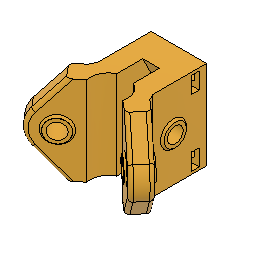
X-Roller v7(1) (Autodesk Fusion 360 design; units mm, degrees)
Autodesk Fusion 360 part; units mm, degrees
note: some values were not read from the file. Chosen so that the rebuilt part matches the saved one: a direction.
sketch "Sketch2" plane through (0, 0, 0) normal (0, 1, 0) x (1, 0, 0) in component "rollers sketches 18mm v10"
  circle A0 centre (0, 0) radius 13.55
  circle A1 centre (0, 0) radius 9.1
  line L0 (0, 0) -> (0, 50) construction
  line L1 (0, 0) -> (38.3022, -32.1394) construction
  line L2 (0, 0) -> (50, 0) construction
  line L3 (0, 0) -> (-38.3022, -32.1394) construction
  line L4 (0, 0) -> (50, 0) construction
  dimension "d20" = 27.1
  dimension "d21" = 18.2
  dimension "d22" = 40
  dimension "d23_1" = 50
  dimension "d24_1" = 140
  dimension "d25_1" = 50
  dimension "d26_1" = 11
  dimension "d27_1" = 11
  dimension "d28_1" = 11
  dimension "d132" = 50
  measures "d20" diameter of A0
  measures "d21" diameter of A1
  measures "d22" angle of L1 L2
  measures "d24_1" angle of L3 L4
  measures "d28_1" distance of A0.centre
sketch "Sketch3" plane through (0, 0, 0) normal (1, 0, 0) x (0, 0, -1) in component "rollers sketches 18mm v10"
  circle A0 centre (20.1, 0) radius 4.2
  circle A1 centre (20.1, 0) radius 11
  circle A2 centre (20.1, 0) radius 6
  circle A3 centre (20.1, 0) radius 13.25
  line L0 (20.1, -13.25) -> (0.1513, -13.25)
  line L1 (20.1, 13.25) -> (0.1513, 13.25)
  line L2 (0.1513, 13.25) -> (0.1513, -13.25)
  line L3 (0.1514, -70) -> (0.1513, 70)
  line L4 (0.1513, 70) -> (31.9687, 5.8904)
  line L5 (0.1514, -70) -> (31.9687, -5.8904)
  dimension "d29_1" = 8.4
  dimension "d30_1" = 22
  dimension "d31_1" = 12
  dimension "d62_1" = 26.5
  dimension "d144" = 70
  dimension "d145" = 70
  measures "d29_1" diameter of A0
  measures "d30_1" diameter of A1
  measures "d31_1" diameter of A2
  measures "d62_1" diameter of A3
ref_plane "WorkPlane1" through (-19.1511, 0, 16.0697) normal (0.642788, 0, 0.766044) x (-0.766044, 0, 0.642788) in component "rollers sketches 18mm v10"
ref_plane "WorkPlane2" through (19.1511, 0, 16.0697) normal (-0.642788, 0, 0.766044) x (0.766044, 0, 0.642788) in component "rollers sketches 18mm v10"
sketch "Sketch4" plane through (-19.1511, 0, 16.0697) normal (0.642788, 0, 0.766044) x (-0.766044, 0, 0.642788) in component "rollers sketches 18mm v10"
  line L0 (23.05, 0) -> (50, 0)
  circle A0 centre (-4.9, 0) radius 4.25
  circle A1 centre (-4.9, 0) radius 6
  circle A2 centre (-4.9, 0) radius 11
  circle A3 centre (-4.9, 0) radius 13.25
  line L1 (-25, 0) -> (-25, 13.25)
  line L2 (-25, 13.25) -> (-4.9, 13.25)
  line L3 (-25, 0) -> (-24.9683, -13.25)
  line L4 (-24.9683, -13.25) -> (-4.9, -13.25)
  line L5 (11.7612, -31.776) -> (-18.2997, -31.776)
  line L6 (-18.2997, -31.776) -> (-18.2997, 33.967)
  line L7 (-18.2997, 33.967) -> (11.7612, 33.967)
  line L8 (11.7612, 33.967) -> (11.7612, -31.776)
  line L9 (-18, 35) -> (-18, -35)
  line L10 (-18, -35) -> (5.0564, -8.7426)
  line L11 (-18, 35) -> (5.0564, 8.7426)
  dimension "d40_1" = 8.5
  dimension "d42_1" = 12
  dimension "d43" = 22
  dimension "d96" = 26.5
  dimension "d139" = 13.25
  dimension "d140" = 13.25
  dimension "d148" = 35
  dimension "d154" = 35
  dimension "d155" = 7
  measures "d40_1" diameter of A0
  measures "d42_1" diameter of A1
  measures "d43" diameter of A2
  measures "d96" diameter of A3
  measures "d139" distance of origin
  measures "d140" distance of origin
  measures "d148" distance of origin
  measures "d154" distance of origin
  measures "d155" distance of L9 origin
sketch "Sketch5" plane through (19.1511, 0, 16.0697) normal (-0.642788, 0, 0.766044) x (0.766044, 0, 0.642788) in component "rollers sketches 18mm v10"
  line L0 (-44.9577, 0) -> (-39.8242, 0)
  circle A0 centre (-4.9, 0) radius 4.25
  circle A1 centre (-4.9, 0) radius 6
  circle A2 centre (-4.9, 0) radius 11
  circle A3 centre (-4.9, 0) radius 13.25
  dimension "d41_1" = 8.5
  dimension "d44" = 12
  dimension "d45" = 22
  dimension "d97" = 26.5
  measures "d41_1" diameter of A0
  measures "d44" diameter of A1
  measures "d45" diameter of A2
  measures "d97" diameter of A3
sketch "Sketch7" plane through (0, 0, 0) normal (0, 1, 0) x (1, 0, 0) in component "rollers sketches 18mm v10"
  circle A0 centre (0, 0) radius 10
  circle A1 centre (0, 0) radius 13.55
  line L0 (0, 9.1) -> (0, 31.1)
  line L1 (-15, 9.0139) -> (-15, 38)
  line L2 (-15, 38) -> (15, 38)
  line L3 (15, 38) -> (15, 9.0139)
  line L4 (-5.1, 9.0139) -> (-15, 9.0139)
  line L5 (5.1, 9.0139) -> (15, 9.0139)
  line L6 (-15, 9.0139) -> (15, 9.0139)
  line L7 (0, 0) -> (0, 50)
  line L8 (-15, 0) -> (-15, 54) construction
  line L9 (0, 0) -> (50, 0)
  line L10 (0, 0) -> (38.3022, -32.1394)
  line L11 (6.7412, -5.6565) -> (16.383, 5.8341)
  line L12 (16.383, 5.8341) -> (35.1894, -9.9463)
  line L13 (35.1894, -9.9463) -> (25.5476, -21.437)
  circle A2 centre (0, 0) radius 17.5
  line L14 (-23.824, -19.9907) -> (-6.971, -5.8494)
  line L15 (-6.0078, -5.0411) -> (-15.6496, 6.4495)
  line L16 (-15.6496, 6.4495) -> (-35.1894, -9.9463)
  line L17 (-36.8084, -30.8859) -> (-57.4533, -48.2091)
  line L18 (0, 0) -> (-38.3022, -32.1394)
  line L19 (-35.1894, -9.9463) -> (-25.5476, -21.437)
  line L20 (-28.5687, -17.8366) -> (-9.7827, -2.0733)
  line L21 (-25.5476, -21.437) -> (-5.2474, -4.4031)
  line L22 (28.5687, -17.8366) -> (9.7827, -2.0733)
  line L23 (5.2474, -4.4031) -> (25.5476, -21.437)
  dimension "d85_1" = 30
  dimension "d86_1" = 15
  dimension "d89_1" = 8.8
  dimension "d91_1" = 15
  dimension "d95" = 15
  dimension "d98" = 4.7
  dimension "d99_1" = 4.7
  dimension "d120" = 35
  dimension "d149" = 20
  dimension "d134" = 38
  measures "d86_1" distance of L1 L7
  measures "d89_1" distance of A0.centre
  measures "d91_1" distance of A0.centre
  measures "d95" distance of A0.centre
  measures "d98" distance of L20 L21
  measures "d99_1" distance of L22 L23
  measures "d120" diameter of A2
  measures "d149" diameter of A0
  measures "d134" distance of L2 A0.centre
ref_plane "WorkPlane5" through (0, 0, -38) normal (0, 0, 1) x (1, 0, 0) in component "rollers sketches 18mm v10"
sketch "Sketch9" plane through (0, 0, -38) normal (0, 0, 1) x (1, 0, 0) in component "rollers sketches 18mm v10"
  circle A0 centre (-10.5, 36) radius 2.25
  circle A1 centre (10.5, 36) radius 2.25
  circle A2 centre (-10.5, -18) radius 2.25
  circle A3 centre (-10.5, -36) radius 2.25
  circle A4 centre (10.5, 18) radius 2.25
  circle A5 centre (10.5, -36) radius 2.25
  circle A6 centre (10.5, -18) radius 2.25
  circle A7 centre (-10.5, 18) radius 2.25
  line L0 (-15, -24) -> (-15, 24)
  line L1 (-10.5, -54) -> (-10.5, -6.4658) construction
  line L2 (-10.5, -16) -> (-10.5, 31.5342) construction
  line L3 (0, 24) -> (15, 24)
  line L4 (10.5, -36) -> (10.5, 11.5342) construction
  line L5 (-10.5, -36) -> (-10.5, 11.5342) construction
  line L6 (10.5, -18) -> (10.5, 29.5342) construction
  line L7 (-10.5, -18) -> (-10.5, 29.5342) construction
  line L8 (15, -24) -> (0, -24)
  line L9 (15, 24) -> (15, -24)
  line L10 (0, 24) -> (0, -24)
  line L11 (-15, 24) -> (0, 24)
  line L12 (-15, -24) -> (0, -24)
  line L13 (10.5, 0) -> (10.5, 47.5342) construction
  line L14 (10.5, -54) -> (10.5, -6.4658) construction
  line L15 (-15, 0) -> (15, 0)
  dimension "d146" = 4.5
  dimension "d147" = 4.5
  dimension "d172" = 24
  dimension "d173" = 18
  dimension "d174" = 18
  dimension "d175" = 18
  dimension "d176" = 18
  dimension "d177" = 48
  dimension "d178" = 18
  dimension "d179" = 18
  dimension "d180" = 18
  dimension "d181" = 18
  measures "d146" diameter of A0
  measures "d147" distance of L0 L2
  measures "d172" distance of L3 L15
  measures "d173" distance of origin
  measures "d175" distance of origin
  measures "d178" distance of origin
  measures "d179" distance of origin
extrude "Extrude16" add sketch "Sketch7" along normal mid plane 48 contours A0 A1 L0 L4 L6 L7 | A0 A1 L4 L6 L15 | A1 L0 L4 L6 L7 A2 | A0 A1 L15 L20 | A1 L4 L6 A2 L15 L16 | L0 L1 L2 L7 A2 | A1 A2 L15 L16 L20 | A2 L16 L19 L20 makes body 1 in component "rollers sketches 18mm v10"
extrude "Extrude17" cut sketch "Sketch4" against normal blind 31 contours A0 bodies 1 in component "rollers sketches 18mm v10"
extrude "Extrude21" add sketch "Sketch4" against normal blind 16 contours A1 bodies 1 in component "rollers sketches 18mm v10"
extrude "Extrude22" cut sketch "Sketch4" against normal blind 3.5 contours A1 bodies 1 in component "rollers sketches 18mm v10"
extrude "Extrude23" cut sketch "Sketch3" along normal mid plane 58 contours A0 bodies 1 in component "rollers sketches 18mm v10"
extrude "Extrude24" cut sketch "Sketch3" along normal mid plane 9 contours A1 | A3 | A3 L1 L3 L4 | A3 L0 L3 L5 | A3 L0 L1 L2 L3 bodies 1 in component "rollers sketches 18mm v10"
extrude "Extrude25" add sketch "Sketch3" against normal blind 16 contours A2 bodies 1 in component "rollers sketches 18mm v10"
extrude "Extrude26" cut sketch "Sketch3" along normal mid plane 7 contours A2 bodies 1 in component "rollers sketches 18mm v10"
extrude "Extrude27" cut sketch "Sketch4" against normal blind 31 contours A3 L5 L7 L8 L10 L11 bodies 1 in component "rollers sketches 18mm v10"
sketch "Sketch9 (2)" plane through (-15, 0, 0) normal (-1, 0, 0) x (0, 0, 1)
  circle A0 centre (-20.1, 0) radius 6
  line L0 (-9.0139, -24) -> (-9.0139, 24)
  line L1 (-9.0139, 24) -> (-38, 24)
  line L2 (-38, 24) -> (-38, -24)
  line L3 (-38, -24) -> (-9.0139, -24)
  line L4 (-47.8567, 18) -> (-16.3238, 18) construction
  line L5 (-52.0724, -18) -> (-19.1904, -18) construction
  line L6 (-30, 13.5) -> (-34, 13.5)
  line L7 (-34, 13.5) -> (-34, 22.5)
  line L8 (-34, 22.5) -> (-30, 22.5)
  line L9 (-30, 22.5) -> (-30, 13.5)
  line L10 (-30, 13.5) -> (-34, 22.5) construction
  line L11 (-34, 13.5) -> (-30, 22.5) construction
  line L12 (-38, -24) -> (-38, 24)
  line L13 (-34, -13.5) -> (-30, -13.5)
  line L14 (-30, -13.5) -> (-30, -22.5)
  line L15 (-30, -22.5) -> (-34, -22.5)
  line L16 (-34, -22.5) -> (-34, -13.5)
  line L17 (-34, -13.5) -> (-30, -22.5) construction
  line L18 (-30, -13.5) -> (-34, -22.5) construction
  dimension "d156" = 4
  dimension "d157" = 4
  dimension "d158" = 9
  dimension "d159" = 4
  dimension "d182" = 4
  dimension "d183" = 9
  measures "d156" distance of L7 L12
  measures "d158" distance of origin
  measures "d159" distance of L12 L16
  measures "d183" distance of origin
extrude "Extrude28" cut sketch "Sketch9 (2)" against normal blind 10 contours L6 L7 L8 L9 | L13 L14 L15 L16 bodies 1 in component "rollers sketches 18mm v10"
extrude "Extrude29" cut sketch "Sketch9" along normal blind 12 contours A2 | A7 bodies 1 in component "rollers sketches 18mm v10"
fillet "Fillet6" radius 2 6 edges at (-27.5348, -16.3713, 3.5234) (-35.1894, 0, 9.9463) (-27.5348, 16.3713, 3.5234) (-20.9141, 16.3713, 11.4136) (-28.5687, 0, 17.8366) (-20.9141, -16.3713, 11.4136) on bodies 1 in component "rollers sketches 18mm v10"
chamfer "Chamfer3" distance 1 angle 45 4 edges at (-20.7541, 2.1697, -2.1664) (-15, -2.1697, -14.506) (-14.1334, -2.1697, 5.7239) (-4.5, -2.1697, -14.506) on bodies 1 in component "rollers sketches 18mm v10"
copy_body "Body->Comp1" bodies 1 removing the originals makes body 2 in component "XRoller alternative US"
mirror "Mirror1" about plane through (0, 0, -10) normal (1, 0, 0) of bodies 2 makes body 3 in component "XRoller alternative US"
combine "Combine1" operation add target body 2 tool bodies 3 in component "XRoller alternative US"
component "rollers sketches 18mm v10" placed x (1, 0, 0) y (0, 1, 0) z (0, 0, 1) at (0, 0, 0)
component "XRoller alternative US" placed x (1, 0, 0) y (0, 1, 0) z (0, 0, 1) at (0, 0, 0) in component "rollers sketches 18mm v10"
equation "d20 = PipeDiameter + 9.3 mm"
equation "d21 = PipeDiameter + 0.4 mm"
equation "d26_1 = BallBearingRadius"
equation "d27_1 = BallBearingRadius"
equation "d28_1 = BallBearingRadius"
equation "d29_1 = BallBInternalR * 2 + 0.4 mm"
equation "d30_1 = BallBearingRadius * 2"
equation "d31_1 = BallBInternalR * 2 + 4 mm"
equation "d40_1 = BallBInternalR * 2 + 0.5 mm"
equation "d42_1 = BallBInternalR * 2 + 4 mm"
equation "d43 = BallBearingRadius * 2"
equation "d62_1 = BallBearingRadius * 2 + 4.5 mm"
equation "d96 = BallBearingRadius * 2 + 4.5 mm"
equation "d120 = PipeDiameter + 17.2 mm"
equation "d149 = PipeDiameter + 2.2 mm"
equation "PipeDiameter = 17.8 mm"
equation "BallBearingRadius = 11 mm"
equation "BallBInternalR = 4 mm"
equation "d132 = BallBearingRadius * 2 + PipeDiameter / 2 + 19.1 mm"
equation "d134 = PipeDiameter / 2 + BallBearingRadius * 2 + 7.1 mm"
equation "d139 = ( BallBearingRadius * 2 + 4.5 mm ) / 2"
equation "d140 = ( BallBearingRadius * 2 + 4.5 mm ) / 2"
